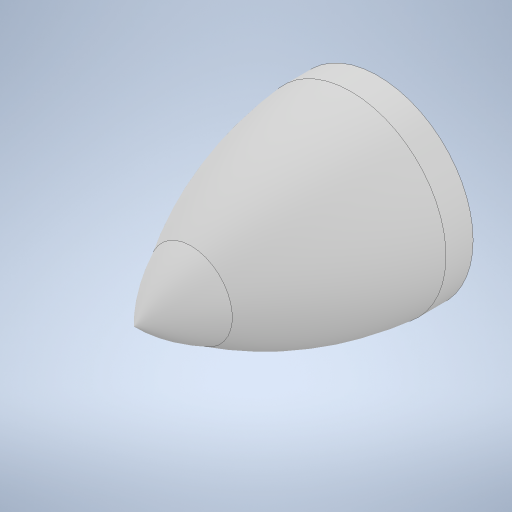
# Autodesk Inventor part: ex_tank_O
Saved by Autodesk Inventor 2024 (Build 280153000, 153)
## iProperties
Created: 2023-06-07
Part Number: ex_tank_O
Material: Generic
Document SubType Name: Modeling
Designer: tamiz
Density: 1 g/cm^3
Appearance: Default
Author: tamiz
Autodesk Inventor part; units mm, degrees
ref_plane "YZ Plane" through (0, 0, 0) normal (1, 0, 0) x (0, 1, 0)
ref_plane "XZ Plane" through (0, 0, 0) normal (0, 1, 0) x (-1, 0, 0)
ref_plane "XY Plane" through (0, 0, 0) normal (0, 0, 1) x (1, 0, 0)
sketch "Sketch1" plane through (0, 0, 0) normal (0, 0, 1) x (1, 0, 0)
  circle A0 centre (0, 0) radius 5334
  dimension "d0" = 10668
  constraints: 1 centre point, 1 coincident
  measures "d0" diameter of A0
extrude "Extrusion1" add sketch "Sketch1" against normal blind 1524
sketch "Sketch5" plane through (0, 0, 0) normal (0, 0, 1) x (1, 0, 0)
  circle A0 centre (0, 0) radius 4876.8
  constraints: 1 centre point, 1 coincident
extrude "Extrusion4" cut sketch "Sketch5" against normal blind 1066.8
sketch "Sketch6" plane through (0, 0, 0) normal (1, 0, 0) x (0, 1, 0)
  arc A0 (2323.259, 8987.0596) -> (0, 12192) centre (-7746.6179, 4131.9476) ccw
  arc A1 (5334, 0) -> (2323.259, 8987.0596) centre (-14818.0717, -1753.2728) ccw
  arc A2 (4875.0327, 0) -> (1922.3284, 8765.8209) centre (-14818.0717, -1753.2728) ccw
  arc A3 (1922.3284, 8765.8209) -> (0, 11544.8563) centre (-7746.6179, 4131.9476) ccw
  line L0 (5334, 0) -> (-5334, 0) projected
  line L1 (5334, 0) -> (4875.0327, 0)
  line L2 (0, 11544.8563) -> (0, 12192)
  line L3 (0, 0) -> (0, 15930.1322) construction
  point P0 (4875.0327, 0)
  dimension "d19" = 457.2
  constraints: 8 point on circle, 6 end point, 4 centre point, 2 vertical
  measures "d19" radial gap between concentric circles of A1 A2
revolve "Revolution2" add sketch "Sketch6" angle 360 about axis through (0, 0, 0) along (0, 0, 1)
body "Solid1"
